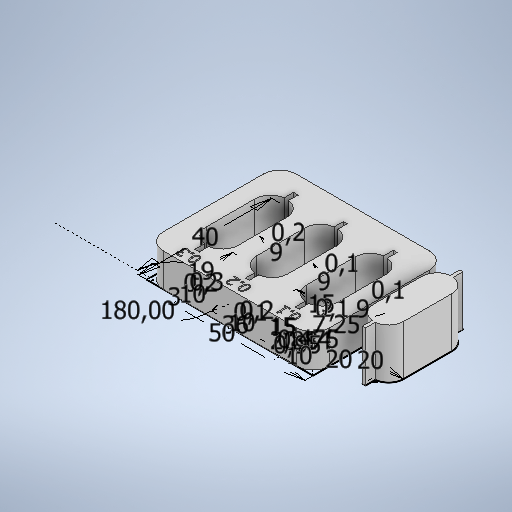
# Autodesk Inventor part: test_servo_syze
Saved by Autodesk Inventor 2025 (Build 290162000, 162)
## iProperties
Created: 2026-07-25
Part Number: test_servo_syze
Material: Типовые
Document SubType Name: Modeling
Designer: garin
Density: 1 g/cm^3
Appearance: По умолчанию
Author: garin
Autodesk Inventor part; units mm, degrees
ref_plane "YZ Plane" through (0, 0, 0) normal (1, 0, 0) x (0, 1, 0)
ref_plane "XZ Plane" through (0, 0, 0) normal (0, 1, 0) x (-1, 0, 0)
ref_plane "XY Plane" through (0, 0, 0) normal (0, 0, 1) x (1, 0, 0)
sketch "Эскиз1" plane through (0, 0, 0) normal (0, 1, 0) x (-1, 0, 0)
  line L0 (0, 0) -> (0, 7.25) construction
  line L1 (0, 0) -> (5.326, 0) construction
  line L2 (0, 0) -> (0, -7.25) construction
  line L3 (0, 7.25) -> (0, -7.25) construction
  line L4 (-4.5, 7.25) -> (-4.5, -7.25)
  line L5 (4.5, -7.25) -> (4.5, 7.25)
  arc A0 (4.5, 7.25) -> (-4.5, 7.25) centre (0, 7.25) ccw
  arc A1 (-4.5, -7.25) -> (4.5, -7.25) centre (0, -7.25) ccw
  line L6 (4.6, 7.25) -> (4.6, -7.25)
  arc A2 (-4.6, -7.25) -> (4.6, -7.25) centre (0, -7.25) ccw
  line L7 (-4.6, -7.25) -> (-4.6, 7.25)
  arc A3 (4.6, 7.25) -> (-4.6, 7.25) centre (0, 7.25) ccw
  line L8 (4.6, 0) -> (6.6, 0) construction
  line L9 (15, 0) -> (15, 7.25) construction
  line L10 (15, 0) -> (15, -7.25) construction
  line L11 (30, 0) -> (30, 7.25) construction
  line L12 (30, 0) -> (30, -7.25) construction
  line L13 (30, 7.25) -> (30, -7.25) construction
  line L14 (25.5, 7.25) -> (25.5, -7.25)
  line L15 (34.5, -7.25) -> (34.5, 7.25)
  arc A4 (34.5, 7.25) -> (25.5, 7.25) centre (30, 7.25) ccw
  arc A5 (25.5, -7.25) -> (34.5, -7.25) centre (30, -7.25) ccw
  line L16 (15, 7.25) -> (15, -7.25) construction
  line L17 (10.5, 7.25) -> (10.5, -7.25)
  line L18 (19.5, -7.25) -> (19.5, 7.25)
  arc A6 (19.5, 7.25) -> (10.5, 7.25) centre (15, 7.25) ccw
  arc A7 (10.5, -7.25) -> (19.5, -7.25) centre (15, -7.25) ccw
  line L19 (25.2, 7.25) -> (25.2, -7.25)
  arc A8 (25.2, -7.25) -> (34.8, -7.25) centre (30, -7.25) ccw
  line L20 (34.8, -7.25) -> (34.8, 7.25)
  arc A9 (34.8, 7.25) -> (25.2, 7.25) centre (30, 7.25) ccw
  line L21 (10.3, 7.25) -> (10.3, -7.25)
  arc A10 (10.3, -7.25) -> (19.7, -7.25) centre (15, -7.25) ccw
  line L22 (19.7, -7.25) -> (19.7, 7.25)
  arc A11 (19.7, 7.25) -> (10.3, 7.25) centre (15, 7.25) ccw
  line L23 (0, 11.75) -> (0, 21.75) construction
  line L24 (15, 11.75) -> (15, 21.75) construction
  line L25 (30, 11.75) -> (30, 21.75) construction
  line L26 (27.0849, 19) -> (33, 19) construction
  line L27 (33, 19) -> (33, 15.7607) construction
  line L28 (33, 15.7607) -> (27.0849, 15.7607) construction
  line L29 (27.0849, 15.7607) -> (27.0849, 19) construction
  line L30 (-10, -20) -> (40, -20)
  line L31 (40, -20) -> (40, 20)
  line L32 (40, 20) -> (-10, 20)
  line L33 (-10, 20) -> (-10, -20)
  line L34 (-10, -20) -> (40, 20) construction
  line L35 (40, -20) -> (-10, 20) construction
  line L36 (-24.5, 7.25) -> (-24.5, -7.25)
  arc A12 (-24.5, -7.25) -> (-15.5, -7.25) centre (-20, -7.25) ccw
  line L37 (-15.5, -7.25) -> (-15.5, 7.25)
  arc A13 (-15.5, 7.25) -> (-24.5, 7.25) centre (-20, 7.25) ccw
  line L38 (30, 0) -> (33, 0) construction
  line L39 (33, 0) -> (33, 19) construction
  line L40 (33, 19) -> (30, 19) construction
  line L41 (30, 19) -> (30, 0) construction
  line L42 (0, 11.75) -> (-0.475, 11.75) construction
  line L43 (15, 11.75) -> (14.525, 11.75) construction
  line L44 (30, 11.75) -> (29.525, 11.75) construction
  line L45 (-0.475, 11.75) -> (0.475, 11.75)
  line L46 (0.475, 11.75) -> (0.475, 14.634)
  line L47 (0.475, 14.634) -> (-0.475, 14.634)
  line L48 (-0.475, 14.634) -> (-0.475, 11.75)
  line L49 (0.475, 11.75) -> (0.475, 11.7249)
  line L50 (-0.475, 11.75) -> (-0.475, 11.7249)
  line L51 (14.525, 11.75) -> (14.525, 11.7249)
  line L52 (14.525, 14.634) -> (14.525, 11.75)
  line L53 (15.475, 14.634) -> (14.525, 14.634)
  line L54 (15.475, 11.75) -> (15.475, 14.634)
  line L55 (15.475, 11.75) -> (15.475, 11.7249)
  line L56 (29.525, 11.75) -> (29.525, 11.7249)
  line L57 (29.525, 14.634) -> (29.525, 11.75)
  line L58 (30.475, 14.634) -> (29.525, 14.634)
  line L59 (30.475, 11.75) -> (30.475, 14.634)
  line L60 (30.475, 11.75) -> (30.475, 11.7249)
  line L61 (0.475, -11.75) -> (0.475, -14.634)
  line L62 (0.475, -14.634) -> (-0.475, -14.634)
  line L63 (-0.475, -14.634) -> (-0.475, -11.75)
  line L64 (0.475, -11.75) -> (0.475, -11.7249)
  line L65 (-0.475, -11.75) -> (-0.475, -11.7249)
  line L66 (14.525, -11.75) -> (14.525, -11.7249)
  line L67 (14.525, -14.634) -> (14.525, -11.75)
  line L68 (15.475, -14.634) -> (14.525, -14.634)
  line L69 (15.475, -11.75) -> (15.475, -14.634)
  line L70 (15.475, -11.75) -> (15.475, -11.7249)
  line L71 (29.525, -11.75) -> (29.525, -11.7249)
  line L72 (29.525, -14.634) -> (29.525, -11.75)
  line L73 (30.475, -14.634) -> (29.525, -14.634)
  line L74 (30.475, -11.75) -> (30.475, -14.634)
  line L75 (30.475, -11.75) -> (30.475, -11.7249)
  line L76 (29.325, 11.7249) -> (29.325, 11.75)
  line L77 (29.325, 11.75) -> (29.325, 14.834)
  line L78 (29.325, 14.834) -> (30.675, 14.834)
  line L79 (30.675, 14.834) -> (30.675, 11.75)
  line L80 (30.675, 11.75) -> (30.675, 11.7249)
  line L81 (30.675, 11.7249) -> (30.675, 11.6991)
  line L82 (29.325, 11.7249) -> (29.325, 11.6991)
  line L83 (29.325, -11.7249) -> (29.325, -11.75)
  line L84 (29.325, -11.75) -> (29.325, -14.834)
  line L85 (29.325, -14.834) -> (30.675, -14.834)
  line L86 (30.675, -14.834) -> (30.675, -11.75)
  line L87 (30.675, -11.75) -> (30.675, -11.7249)
  line L88 (30.675, -11.7249) -> (30.675, -11.6991)
  line L89 (29.325, -11.7249) -> (29.325, -11.6991)
  line L90 (14.425, -11.7249) -> (14.425, -11.75)
  line L91 (14.425, -11.75) -> (14.425, -14.734)
  line L92 (14.425, -14.734) -> (15.575, -14.734)
  line L93 (15.575, -14.734) -> (15.575, -11.75)
  line L94 (15.575, -11.75) -> (15.575, -11.7249)
  line L95 (15.575, -11.7249) -> (15.575, -11.7131)
  line L96 (14.425, -11.7249) -> (14.425, -11.7131)
  line L97 (14.425, 11.7249) -> (14.425, 11.75)
  line L98 (14.425, 11.75) -> (14.425, 14.734)
  line L99 (14.425, 14.734) -> (15.575, 14.734)
  line L100 (15.575, 14.734) -> (15.575, 11.75)
  line L101 (15.575, 11.75) -> (15.575, 11.7249)
  line L102 (15.575, 11.7249) -> (15.575, 11.7131)
  line L103 (14.425, 11.7249) -> (14.425, 11.7131)
  line L104 (-0.575, -11.7249) -> (-0.575, -11.75)
  line L105 (-0.575, -11.75) -> (-0.575, -14.734)
  line L106 (-0.575, -14.734) -> (0.575, -14.734)
  line L107 (0.575, -14.734) -> (0.575, -11.75)
  line L108 (0.575, -11.75) -> (0.575, -11.7249)
  line L109 (0.575, -11.7249) -> (0.575, -11.7131)
  line L110 (-0.575, -11.7249) -> (-0.575, -11.7131)
  line L111 (0.575, 11.75) -> (0.575, 14.734)
  line L112 (0.575, 14.734) -> (-0.575, 14.734)
  line L113 (-0.575, 14.734) -> (-0.575, 11.75)
  line L114 (0.575, 11.75) -> (0.575, 11.7131)
  line L115 (-0.575, 11.75) -> (-0.575, 11.7131)
  line L116 (-19.525, 11.75) -> (-19.525, 14.634)
  line L117 (-19.525, 14.634) -> (-20.475, 14.634)
  line L118 (-20.475, 14.634) -> (-20.475, 11.75)
  line L119 (-20.475, 11.75) -> (-20.475, 11.7249)
  line L120 (-19.525, 11.75) -> (-19.525, 11.7249)
  line L121 (-19.525, -14.634) -> (-20.475, -14.634)
  line L122 (-20.475, -14.634) -> (-20.475, -11.75)
  line L123 (-19.525, -11.75) -> (-19.525, -14.634)
  line L124 (-19.525, -11.75) -> (-19.525, -11.7249)
  line L125 (-20.475, -11.75) -> (-20.475, -11.7249)
  line L126 (12.0894, 19) -> (18.0045, 19) construction
  line L127 (18.0045, 19) -> (18.0045, 15.7607) construction
  line L128 (18.0045, 15.7607) -> (12.0894, 15.7607) construction
  line L129 (12.0894, 15.7607) -> (12.0894, 19) construction
  line L130 (-3, 15.7607) -> (-3, 19) construction
  line L131 (-3, 19) -> (2.9151, 19) construction
  line L132 (2.9151, 19) -> (2.9151, 15.7607) construction
  line L133 (2.9151, 15.7607) -> (-3, 15.7607) construction
  line L134 (33, 19) -> (-3, 19) construction
  line L135 (33, 19) -> (69, 19) construction
  spline S0 degree 2 poles (29.2042, 17.4118) (29.2042, 16.5917) (28.7275, 15.8236) (28.231, 15.8236) knots 0 0 0 1 2 2 2
  spline S1 degree 2 poles (28.231, 15.8236) (27.7271, 15.8236) (27.2554, 16.6066) (27.2554, 17.4093) knots 0 0 0 1 2 2 2
  spline S2 degree 2 poles (27.2554, 17.4093) (27.2554, 18.2343) (27.7321, 18.9975) (28.231, 18.9975) knots 0 0 0 1 2 2 2
  spline S3 degree 2 poles (28.231, 18.9975) (28.7324, 18.9975) (29.2042, 18.2071) (29.2042, 17.4118) knots 0 0 0 1 2 2 2
  spline S4 degree 2 poles (28.6806, 16.4831) (28.7398, 16.6337) (28.7892, 17.0981) (28.7892, 17.4118) knots 0 0 0 1 2 2 2
  spline S5 degree 2 poles (28.7892, 17.4118) (28.7892, 17.7255) (28.7398, 18.1874) (28.6781, 18.343) knots 0 0 0 1 2 2 2
  spline S6 degree 2 poles (28.6781, 18.343) (28.6163, 18.4986) (28.4014, 18.6591) (28.231, 18.6591) knots 0 0 0 1 2 2 2
  spline S7 degree 2 poles (28.231, 18.6591) (28.0606, 18.6591) (27.8408, 18.4986) (27.7765, 18.338) knots 0 0 0 1 2 2 2
  spline S8 degree 2 poles (27.7765, 18.338) (27.7148, 18.1824) (27.6703, 17.7082) (27.6703, 17.4093) knots 0 0 0 1 2 2 2
  spline S9 degree 2 poles (27.6703, 17.4093) (27.6703, 17.0882) (27.7098, 16.6584) (27.7741, 16.4905) knots 0 0 0 1 2 2 2
  spline S10 degree 2 poles (27.7741, 16.4905) (27.8333, 16.3324) (28.0532, 16.162) (28.231, 16.162) knots 0 0 0 1 2 2 2
  spline S11 degree 2 poles (28.231, 16.162) (28.399, 16.162) (28.6188, 16.3225) (28.6806, 16.4831) knots 0 0 0 1 2 2 2
  line L136 (30.249, 15.8878) -> (29.76, 15.8878)
  line L137 (29.76, 15.8878) -> (29.76, 16.4707)
  line L138 (29.76, 16.4707) -> (30.249, 16.4707)
  line L139 (30.249, 16.4707) -> (30.249, 15.8878)
  spline S12 degree 2 poles (31.6866, 18.6468) (31.5754, 18.6468) (31.3556, 18.5924) (31.2494, 18.5505) knots 0 0 0 1 2 2 2
  spline S13 degree 2 poles (31.2494, 18.5505) (31.1506, 18.5085) (31.0048, 18.4195) (30.948, 18.38) knots 0 0 0 1 2 2 2
  line L140 (30.948, 18.38) -> (30.9233, 18.38)
  line L141 (30.9233, 18.38) -> (30.9233, 18.8123)
  spline S14 degree 2 poles (30.9233, 18.8123) (31.0567, 18.8839) (31.5137, 19) (31.7187, 19) knots 0 0 0 1 2 2 2
  spline S15 degree 2 poles (31.7187, 19) (31.9262, 19) (32.2349, 18.916) (32.3609, 18.8271) knots 0 0 0 1 2 2 2
  spline S16 degree 2 poles (32.3609, 18.8271) (32.4943, 18.7308) (32.6326, 18.4517) (32.6326, 18.2639) knots 0 0 0 1 2 2 2
  spline S17 degree 2 poles (32.6326, 18.2639) (32.6326, 18.012) (32.3016, 17.6316) (32.0694, 17.5822) knots 0 0 0 1 2 2 2
  line L142 (32.0694, 17.5822) -> (32.0694, 17.5526)
  spline S18 degree 2 poles (32.0694, 17.5526) (32.1658, 17.5328) (32.3856, 17.4439) (32.4794, 17.355) knots 0 0 0 1 2 2 2
  spline S19 degree 2 poles (32.4794, 17.355) (32.5733, 17.2685) (32.6919, 16.9919) (32.6919, 16.7918) knots 0 0 0 1 2 2 2
  spline S20 degree 2 poles (32.6919, 16.7918) (32.6919, 16.5868) (32.5511, 16.2385) (32.4226, 16.1051) knots 0 0 0 1 2 2 2
  spline S21 degree 2 poles (32.4226, 16.1051) (32.2893, 15.9668) (31.9113, 15.8236) (31.6717, 15.8236) knots 0 0 0 1 2 2 2
  spline S22 degree 2 poles (31.6717, 15.8236) (31.442, 15.8236) (30.9925, 15.9347) (30.8394, 16.0113) knots 0 0 0 1 2 2 2
  line L143 (30.8394, 16.0113) -> (30.8394, 16.4435)
  line L144 (30.8394, 16.4435) -> (30.869, 16.4435)
  spline S23 degree 2 poles (30.869, 16.4435) (30.9974, 16.3497) (31.4322, 16.1768) (31.647, 16.1768) knots 0 0 0 1 2 2 2
  spline S24 degree 2 poles (31.647, 16.1768) (31.773, 16.1768) (32.025, 16.2558) (32.1089, 16.3472) knots 0 0 0 1 2 2 2
  spline S25 degree 2 poles (32.1089, 16.3472) (32.1905, 16.4386) (32.2769, 16.656) (32.2769, 16.8214) knots 0 0 0 1 2 2 2
  spline S26 degree 2 poles (32.2769, 16.8214) (32.2769, 16.9869) (32.1806, 17.2018) (32.0941, 17.2636) knots 0 0 0 1 2 2 2
  spline S27 degree 2 poles (32.0941, 17.2636) (32.0077, 17.3253) (31.773, 17.3723) (31.6347, 17.3723) knots 0 0 0 1 2 2 2
  line L145 (31.6347, 17.3723) -> (31.4618, 17.3723)
  line L146 (31.4618, 17.3723) -> (31.4618, 17.7107)
  line L147 (31.4618, 17.7107) -> (31.5976, 17.7107)
  spline S28 degree 2 poles (31.5976, 17.7107) (31.8718, 17.7107) (32.2176, 17.9725) (32.2176, 18.2219) knots 0 0 0 1 2 2 2
  spline S29 degree 2 poles (32.2176, 18.2219) (32.2176, 18.338) (32.1287, 18.5035) (32.0571, 18.5529) knots 0 0 0 1 2 2 2
  spline S30 degree 2 poles (32.0571, 18.5529) (31.9805, 18.6048) (31.7928, 18.6468) (31.6866, 18.6468) knots 0 0 0 1 2 2 2
  spline S31 degree 2 poles (14.2087, 17.4118) (14.2087, 16.5917) (13.732, 15.8236) (13.2355, 15.8236) knots 0 0 0 1 2 2 2
  spline S32 degree 2 poles (13.2355, 15.8236) (12.7316, 15.8236) (12.2599, 16.6066) (12.2599, 17.4093) knots 0 0 0 1 2 2 2
  spline S33 degree 2 poles (12.2599, 17.4093) (12.2599, 18.2343) (12.7366, 18.9975) (13.2355, 18.9975) knots 0 0 0 1 2 2 2
  spline S34 degree 2 poles (13.2355, 18.9975) (13.7369, 18.9975) (14.2087, 18.2071) (14.2087, 17.4118) knots 0 0 0 1 2 2 2
  spline S35 degree 2 poles (13.6851, 16.4831) (13.7444, 16.6337) (13.7938, 17.0981) (13.7938, 17.4118) knots 0 0 0 1 2 2 2
  spline S36 degree 2 poles (13.7938, 17.4118) (13.7938, 17.7255) (13.7444, 18.1874) (13.6826, 18.343) knots 0 0 0 1 2 2 2
  spline S37 degree 2 poles (13.6826, 18.343) (13.6209, 18.4986) (13.406, 18.6591) (13.2355, 18.6591) knots 0 0 0 1 2 2 2
  spline S38 degree 2 poles (13.2355, 18.6591) (13.0651, 18.6591) (12.8453, 18.4986) (12.781, 18.338) knots 0 0 0 1 2 2 2
  spline S39 degree 2 poles (12.781, 18.338) (12.7193, 18.1824) (12.6748, 17.7082) (12.6748, 17.4093) knots 0 0 0 1 2 2 2
  spline S40 degree 2 poles (12.6748, 17.4093) (12.6748, 17.0882) (12.7144, 16.6584) (12.7786, 16.4905) knots 0 0 0 1 2 2 2
  spline S41 degree 2 poles (12.7786, 16.4905) (12.8379, 16.3324) (13.0577, 16.162) (13.2355, 16.162) knots 0 0 0 1 2 2 2
  spline S42 degree 2 poles (13.2355, 16.162) (13.4035, 16.162) (13.6233, 16.3225) (13.6851, 16.4831) knots 0 0 0 1 2 2 2
  line L148 (15.2535, 15.8878) -> (14.7645, 15.8878)
  line L149 (14.7645, 15.8878) -> (14.7645, 16.4707)
  line L150 (14.7645, 16.4707) -> (15.2535, 16.4707)
  line L151 (15.2535, 16.4707) -> (15.2535, 15.8878)
  line L152 (17.7483, 15.8878) -> (15.8686, 15.8878)
  line L153 (15.8686, 15.8878) -> (15.8686, 16.32)
  spline S43 degree 2 poles (15.8686, 16.32) (16.0711, 16.5102) (16.4317, 16.8634) (16.6046, 17.0536) knots 0 0 0 1 2 2 2
  spline S44 degree 2 poles (16.6046, 17.0536) (16.9529, 17.4365) (17.2073, 17.8959) (17.2073, 18.1404) knots 0 0 0 1 2 2 2
  spline S45 degree 2 poles (17.2073, 18.1404) (17.2073, 18.2689) (17.1283, 18.4615) (17.0566, 18.5233) knots 0 0 0 1 2 2 2
  spline S46 degree 2 poles (17.0566, 18.5233) (16.985, 18.585) (16.7973, 18.6468) (16.6837, 18.6468) knots 0 0 0 1 2 2 2
  spline S47 degree 2 poles (16.6837, 18.6468) (16.575, 18.6468) (16.3527, 18.5924) (16.2514, 18.5505) knots 0 0 0 1 2 2 2
  spline S48 degree 2 poles (16.2514, 18.5505) (16.165, 18.5159) (16.0044, 18.4171) (15.955, 18.3825) knots 0 0 0 1 2 2 2
  line L154 (15.955, 18.3825) -> (15.9328, 18.3825)
  line L155 (15.9328, 18.3825) -> (15.9328, 18.8172)
  spline S49 degree 2 poles (15.9328, 18.8172) (16.0588, 18.879) (16.5108, 19) (16.7133, 19) knots 0 0 0 1 2 2 2
  spline S50 degree 2 poles (16.7133, 19) (17.1406, 19) (17.6223, 18.548) (17.6223, 18.1627) knots 0 0 0 1 2 2 2
  spline S51 degree 2 poles (17.6223, 18.1627) (17.6223, 17.9824) (17.5383, 17.681) (17.4642, 17.5526) knots 0 0 0 1 2 2 2
  spline S52 degree 2 poles (17.4642, 17.5526) (17.3901, 17.4192) (17.1752, 17.1574) (17.0566, 17.0314) knots 0 0 0 1 2 2 2
  spline S53 degree 2 poles (17.0566, 17.0314) (16.864, 16.8214) (16.3922, 16.3719) (16.2514, 16.241) knots 0 0 0 1 2 2 2
  line L156 (16.2514, 16.241) -> (17.7483, 16.241)
  line L157 (17.7483, 16.241) -> (17.7483, 15.8878)
  spline S54 degree 2 poles (-0.8807, 17.4142) (-0.8807, 16.5942) (-1.3574, 15.826) (-1.8539, 15.826) knots 0 0 0 1 2 2 2
  spline S55 degree 2 poles (-1.8539, 15.826) (-2.3578, 15.826) (-2.8296, 16.609) (-2.8296, 17.4118) knots 0 0 0 1 2 2 2
  spline S56 degree 2 poles (-2.8296, 17.4118) (-2.8296, 18.2368) (-2.3529, 19) (-1.8539, 19) knots 0 0 0 1 2 2 2
  spline S57 degree 2 poles (-1.8539, 19) (-1.3525, 19) (-0.8807, 18.2096) (-0.8807, 17.4142) knots 0 0 0 1 2 2 2
  spline S58 degree 2 poles (-1.4044, 16.4855) (-1.3451, 16.6362) (-1.2957, 17.1006) (-1.2957, 17.4142) knots 0 0 0 1 2 2 2
  spline S59 degree 2 poles (-1.2957, 17.4142) (-1.2957, 17.7279) (-1.3451, 18.1898) (-1.4068, 18.3454) knots 0 0 0 1 2 2 2
  spline S60 degree 2 poles (-1.4068, 18.3454) (-1.4686, 18.5011) (-1.6835, 18.6616) (-1.8539, 18.6616) knots 0 0 0 1 2 2 2
  spline S61 degree 2 poles (-1.8539, 18.6616) (-2.0243, 18.6616) (-2.2442, 18.5011) (-2.3084, 18.3405) knots 0 0 0 1 2 2 2
  spline S62 degree 2 poles (-2.3084, 18.3405) (-2.3701, 18.1849) (-2.4146, 17.7107) (-2.4146, 17.4118) knots 0 0 0 1 2 2 2
  spline S63 degree 2 poles (-2.4146, 17.4118) (-2.4146, 17.0907) (-2.3751, 16.6609) (-2.3109, 16.4929) knots 0 0 0 1 2 2 2
  spline S64 degree 2 poles (-2.3109, 16.4929) (-2.2516, 16.3349) (-2.0318, 16.1644) (-1.8539, 16.1644) knots 0 0 0 1 2 2 2
  spline S65 degree 2 poles (-1.8539, 16.1644) (-1.686, 16.1644) (-1.4661, 16.325) (-1.4044, 16.4855) knots 0 0 0 1 2 2 2
  line L158 (0.1641, 15.8902) -> (-0.325, 15.8902)
  line L159 (-0.325, 15.8902) -> (-0.325, 16.4732)
  line L160 (-0.325, 16.4732) -> (0.1641, 16.4732)
  line L161 (0.1641, 16.4732) -> (0.1641, 15.8902)
  line L162 (2.5057, 15.8902) -> (1.0187, 15.8902)
  line L163 (1.0187, 15.8902) -> (1.0187, 16.2015)
  line L164 (1.0187, 16.2015) -> (1.572, 16.2015)
  line L165 (1.572, 16.2015) -> (1.572, 18.2442)
  line L166 (1.572, 18.2442) -> (1.0187, 18.2442)
  line L167 (1.0187, 18.2442) -> (1.0187, 18.5233)
  spline S66 degree 2 poles (1.0187, 18.5233) (1.3324, 18.5233) (1.6288, 18.7011) (1.6486, 18.9481) knots 0 0 0 1 2 2 2
  line L168 (1.6486, 18.9481) -> (1.9647, 18.9481)
  line L169 (1.9647, 18.9481) -> (1.9647, 16.2015)
  line L170 (1.9647, 16.2015) -> (2.5057, 16.2015)
  line L171 (2.5057, 16.2015) -> (2.5057, 15.8902)
  point P0 (-20, 11.75)
  point P1 (29.325, 12.0023)
  point P2 (30.675, 12.0023)
  point P3 (30.675, -12.0023)
  point P4 (29.325, -12.0023)
  point P5 (14.425, 11.9147)
  point P6 (15.575, 11.9147)
  point P7 (15.575, -11.9147)
  point P8 (14.425, -11.9147)
  point P9 (0.575, -11.8139)
  point P10 (-0.575, -11.8139)
  point P11 (-0.575, 11.8139)
  point P12 (0.575, 11.8139)
  dimension "d0" = 7.25
  dimension "d1" = 9
  dimension "d2" = 0.1
  dimension "d3" = 2
  dimension "d6" = 15
  dimension "d11" = 9
  dimension "d12" = 9
  dimension "d13" = 0.3
  dimension "d14" = 0.2
  dimension "d15" = 10
  dimension "d16" = 10
  dimension "d17" = 10
  dimension "d18" = 50
  dimension "d19" = 40
  dimension "d22" = 20
  dimension "d27" = 3
  dimension "d28" = 19
  dimension "d37" = 0.475
  dimension "d40" = 15
  dimension "d45" = 0.95
  dimension "d46" = 2.884
  dimension "d49" = 15
  dimension "d54" = 0.2
  dimension "d55" = 0.2
  dimension "d56" = 0.1
  dimension "d57" = 0.1
  dimension "d58" = 0.1
  dimension "d59" = 0.1
  dimension "d62" = 20
  dimension "d67" = 36
  dimension "d68" = 180
  constraints: 254 end point, 45 point on circle, 20 parallel, 19 symmetric about line, 14 centre point, 13 tangent, 11 horizontal, 9 vertical, 6 midpoint, 6 point on line, 3 collinear, 3 perpendicular, 2 coincident, 108 other
  measures "d0" distance of L0.start L0.end
  measures "d1" diameter of A1
  measures "d2" distance between parallel lines of L5 L6
  measures "d3" distance of L8.start L8.end
  measures "d6" distance of L0.start L9.start
  measures "d11" diameter of A5
  measures "d12" diameter of A7
  measures "d13" radial gap between concentric circles of A4 A9
  measures "d14" radial gap between concentric circles of A6 A11
  measures "d15" distance of L23.start L23.end
  measures "d16" distance of L24.start L24.end
  measures "d17" distance of L25.start L25.end
  measures "d18" distance of L32.end L31.end
  measures "d19" distance of L31.end L30.end
  measures "d22" distance of L4.start L36.start
  measures "d27" distance of L40.end L39.end
  measures "d28" distance of L39.end L38.end
  measures "d37" distance of L23.start L42.end
  measures "d40" distance of L23.start L43.start
  measures "d45" distance of L47.end L46.end
  measures "d46" distance of L46.end L45.end
  measures "d49" distance of L42.end L51.start
  measures "d54" distance between parallel lines of L59 L79
  measures "d55" distance between parallel lines of L74 L86
  measures "d56" distance between parallel lines of L67 L91
  measures "d57" distance between parallel lines of L54 L100
  measures "d58" distance between parallel lines of L61 L107
  measures "d59" distance between parallel lines of L46 L111
  measures "d62" distance of L45.end L116.start
  measures "d67" distance of L39.end L134.end
  measures "d68" angle of L135 L134
extrude "Выдавливание1" add sketch "Эскиз1" along normal blind 10 contours L33 L32 L31 L30 | S0 S1 S2 S3 | S11 S10 S9 S8 S7 S6 S5 S4 | L136 L137 L138 L139 | S12 S13 L140 L141 S14 S15 S16 S17 L142 S18 S19 S20 S21 S22 L143 L144 S23 S24 S25 S26 S27 L145 L146 L147 S28 S29 S30 | S31 S32 S33 S34 | S42 S41 S40 S39 S38 S37 S36 S35 | L148 L149 L150 L151 | L152 L153 S43 S44 S45 S46 S47 S48 L154 L155 S49 S50 S51 S52 S53 L156 L157 | S54 S55 S56 S57 | S65 S64 S63 S62 S61 S60 S59 S58 | L158 L159 L160 L161 | L162 L163 L164 L165 L166 L167 S66 L168 L169 L170 L171
extrude "Выдавливание2" add sketch "Эскиз1" along normal blind 15 contours A13 L37 A12 L36 | L119 L118 L117 L116 L120 A13 | A12 L124 L123 L121 L122 L125
extrude "Выдавливание3" cut sketch "Эскиз1" against normal blind 1.5 from surface at 10 contours S0 S1 S2 S3 | L136 L137 L138 L139 | S12 S13 L140 L141 S14 S15 S16 S17 L142 S18 S19 S20 S21 S22 L143 L144 S23 S24 S25 S26 S27 L145 L146 L147 S28 S29 S30 | S31 S32 S33 S34 | L148 L149 L150 L151 | L152 L153 S43 S44 S45 S46 S47 S48 L154 L155 S49 S50 S51 S52 S53 L156 L157 | S54 S55 S56 S57 | L158 L159 L160 L161 | L162 L163 L164 L165 L166 L167 S66 L168 L169 L170 L171
fillet "Сопряжение1" radius 5 4 edges at (10, 5, 20) (-40, 5, 20) (-40, 5, -20) (10, 5, -20)
